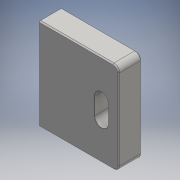
# Autodesk Inventor part: ОПОРА_02
Saved by Autodesk Inventor 2016 (Build 200138000, 138)
## iProperties
Created: 2021-05-03
Part Number: ОПОРА_02
Material: Типовые
Document SubType Name: Modeling
Designer: Лол
Density: 1 g/cm^3
Appearance: По умолчанию
Author: Лол
Autodesk Inventor part; units mm, degrees
ref_plane "YZ Plane" through (0, 0, 0) normal (1, 0, 0) x (0, 1, 0)
ref_plane "XZ Plane" through (0, 0, 0) normal (0, 1, 0) x (-1, 0, 0)
ref_plane "XY Plane" through (0, 0, 0) normal (0, 0, 1) x (1, 0, 0)
sketch "Эскиз1" plane through (0, 0, 0) normal (1, 0, 0) x (0, 1, 0)
  line L0 (-14, 0) -> (14, 0) projected
  line L1 (0, -56) -> (0, 56) projected
  line L2 (10, 40) -> (-10, 40)
  line L3 (-10, 40) -> (-10, -40)
  line L4 (-10, -40) -> (10, -40)
  line L5 (10, -40) -> (10, 40)
  point P0 (0, 0)
  dimension "d0" = 20
  dimension "d1" = 10
  dimension "d2" = 80
  dimension "d3" = 40
  constraints: 8 end point, 2 parallel, 1 horizontal, 1 perpendicular
  measures "d0" distance of L3.end L4.end
  measures "d1" distance between parallel lines of L5 L1
  measures "d2" distance of L2.end L3.end
  measures "d3" distance between parallel lines of L4 L0
extrude "Выдавливание1" add sketch "Эскиз1" against normal blind 70
fillet "Сопряжение1" radius 5 2 edges at (0, 0, 40) (0, 0, -40)
chamfer "Фаска1" distance 1 angle 45 10 edges at (-37.5, 10, 40) (-1.4645, 10, 38.5355) (0, 10, 0) (-1.4645, 10, -38.5355) (-37.5, 10, -40) (-37.5, -10, 40) (-1.4645, -10, 38.5355) (0, -10, 0) (-1.4645, -10, -38.5355) (-37.5, -10, -40)
chamfer "Фаска2" distance 1 angle 45 4 edges at (-70, 10, 0) (-70, 0, 40) (-70, -10, 0) (-70, 0, -40)
sketch "Эскиз3" plane through (-70, 0, 0) normal (-1, 0, 0) x (0, 0, 1)
  line L0 (-56, 0) -> (56, 0) projected
  line L1 (0, 14) -> (0, -14) projected
  circle A0 centre (14, 0) radius 3
  circle A1 centre (-14, 0) radius 3
  dimension "d42" = 6
  dimension "d43" = 6
  dimension "d44" = 28
  dimension "d45" = 14
  constraints: 2 centre point, 2 point on line
  measures "d42" diameter of A0
  measures "d43" diameter of A1
  measures "d44" distance of A1.centre A0.centre
  measures "d45" distance from line of A0.centre L1
hole "Отверстие2" at (-70, 0, 14) at (-70, 0, -14) direction (1, 0, 0) diameter 6 depth 10 tip angle 118 countersink diameter 8 countersink angle 45
sketch "Эскиз4" plane through (-70, 0, 0) normal (-1, 0, 0) x (0, 0, 1)
  line L0 (0, 14) -> (0, -14) projected
  line L1 (-56, 0) -> (56, 0) projected
  circle A0 centre (25, 0) radius 5
  circle A1 centre (-25, 0) radius 5
  point P0 (0, 0)
  dimension "d46" = 10
  dimension "d47" = 50
  dimension "d48" = 25
  constraints: 2 centre point, 2 point on line, 1 equal radius
  measures "d46" diameter of A0
  measures "d47" distance of A1.centre A0.centre
  measures "d48" distance from line of A0.centre L0
hole "Отверстие3" at (-70, 0, 25) at (-70, 0, -25) direction (1, 0, 0) diameter 8.376 depth 31.3 tip angle 118 countersink diameter 13.2 countersink angle 90 thread size "M10x1.5" class "6H" standard "ISO Metric profile"
sketch "Эскиз6" plane through (0, 0, 0) normal (0, 1, 0) x (-1, 0, 0)
  line L0 (-14, 0) -> (84, 0) projected
  line L1 (0, -56) -> (0, 56) projected
  line L2 (70, -39) -> (70, 39) projected
  line L3 (15, 7.5) -> (15, -7.5) construction
  arc A0 (21, 7.5) -> (9, 7.5) centre (15, 7.5) ccw
  arc A1 (9, -7.5) -> (21, -7.5) centre (15, -7.5) ccw
  line L4 (21, 7.5) -> (21, -7.5)
  line L5 (9, 7.5) -> (9, -7.5)
  point P0 (0, 0)
  dimension "d56" = 12
  dimension "d57" = 15
  dimension "d58" = 7.5
  dimension "d59" = 55
  constraints: 6 end point, 4 point on circle, 4 tangent, 2 centre point, 2 coincident, 1 equal radius, 1 vertical
  measures "d56" diameter of A0
  measures "d57" distance of L3.end L3.start
  measures "d58" distance from line of L3.end L0
  measures "d59" distance between parallel lines of L2 L3
extrude "Выдавливание2" cut sketch "Эскиз6" along normal through all both and the other way through all
chamfer "Фаска4" distance 0.2 angle 45 8 edges at (-9, -10, 0) (-15, -10, -13.5) (-21, -10, 0) (-15, -10, 13.5) (-21, 10, 0) (-15, 10, -13.5) (-9, 10, 0) (-15, 10, 13.5)
